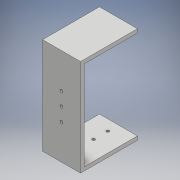
# Autodesk Inventor part: Servo Holder Upper Part
Saved by Autodesk Inventor 2018 (Build 220112000, 112)
## iProperties
Created: 2018-04-22
Part Number: Servo Holder Upper Part
Material: Generic
Document SubType Name: Modeling
Designer: HP
Density: 1 g/cm^3
Appearance: Default
Mass: 3.87293 g
Surface Area: 43.5978 cm^2
Volume: 3.87293 cm^3
Author: HP
Autodesk Inventor part; units mm, degrees
ref_plane "YZ Plane" through (0, 0, 0) normal (1, 0, 0) x (0, 1, 0)
ref_plane "XZ Plane" through (0, 0, 0) normal (0, 1, 0) x (-1, 0, 0)
ref_plane "XY Plane" through (0, 0, 0) normal (0, 0, 1) x (1, 0, 0)
sketch "Sketch9" plane through (0, 0, 0) normal (0, 1, 0) x (-1, 0, 0)
  line L0 (0, 0) -> (-20, 0)
  line L1 (-20, 0) -> (-20, -47)
  line L2 (-20, -47) -> (0, -47)
  line L3 (0, -47) -> (0, 0)
  dimension "d20" = 20
  dimension "d21" = 47
  constraints: 8 end point, 2 parallel, 1 horizontal, 1 perpendicular
  measures "d20" distance of L2.end L1.end
  measures "d21" distance of L1.end L0.end
extrude "Extrusion6" add sketch "Sketch9" along normal blind 2
sketch "Sketch10" plane through (0, 0, 0) normal (0, 0, 1) x (1, 0, 0)
  line L0 (0, 0) -> (20, 0) projected
  line L1 (0, 0) -> (20, 0)
  line L2 (20, 0) -> (20, 30)
  line L3 (20, 30) -> (0, 30)
  line L4 (0, 30) -> (0, 0)
  dimension "d24" = 30
  dimension "d40" = 20
  constraints: 8 end point, 2 parallel, 1 horizontal, 1 perpendicular
  measures "d24" distance of L2.end L1.end
  measures "d40" distance between parallel lines of L2 L4
extrude "Extrusion7" add sketch "Sketch10" along normal blind 2
sketch "Sketch11" plane through (20, 0, -47) normal (0, 0, -1) x (-1, 0, 0)
  line L0 (0, 2) -> (0, 30) projected
  line L1 (0, 0) -> (20, 0) projected
  line L2 (0, 30) -> (20, 30)
  line L3 (20, 30) -> (20, 0)
  line L4 (20, 0) -> (0, 0)
  line L5 (0, 0) -> (0, 30)
  dimension "d39" = 30
  constraints: 8 end point, 2 parallel, 1 horizontal, 1 perpendicular
  measures "d39" distance between parallel lines of L2 L1
extrude "Extrusion8" add sketch "Sketch11" along normal blind 2
sketch "Sketch12" plane through (20, 0, -49) normal (0, 0, -1) x (-1, 0, 0)
  circle A0 centre (10, 24.36) radius 0.75
  line L0 (20, 30) -> (0, 30) projected
  line L1 (0, 30) -> (0, 0) projected
  point P0 (20, 0)
  dimension "d29" = 1.5
  dimension "d30" = 5.64
  dimension "d31" = 10
  constraints: 1 centre point
  measures "d29" diameter of A0
  measures "d30" distance from line of L0 A0.centre
  measures "d31" distance from line of L1 A0.centre
extrude "Extrusion9" cut sketch "Sketch12" against normal blind 2
sketch "Sketch13" plane through (20, 0, -49) normal (0, 0, -1) x (-1, 0, 0)
  circle A0 centre (10, 16.86) radius 0.75
  line L0 (0, 30) -> (0, 0) projected
  circle A1 centre (10, 24.36) radius 0.75 projected
  point P0 (20, 0)
  dimension "d34" = 1.5
  dimension "d35" = 10
  dimension "d36" = 7.5
  constraints: 1 centre point
  measures "d34" diameter of A0
  measures "d35" distance from line of L0 A0.centre
  measures "d36" distance of A1.centre A0.centre
extrude "Extrusion10" cut sketch "Sketch13" against normal blind 2 contours A0
sketch "Sketch14" plane through (0, 0, 0) normal (0, -1, 0) x (1, 0, 0)
  circle A0 centre (10, -23.5) radius 0.75
  line L0 (0, 2) -> (0, -49) projected
  line L1 (20, -47) -> (0, -47) projected
  circle A1 centre (10, -30.6) radius 0.75
  circle A2 centre (10, -16.4) radius 0.75
  point P0 (0, 0)
  dimension "d41" = 1.5
  dimension "d42" = 10
  dimension "d43" = 23.5
  dimension "d44" = 1.5
  dimension "d45" = 7.1
  dimension "d46" = 1.5
  dimension "d47" = 7.1
  constraints: 3 centre point
  measures "d41" diameter of A0
  measures "d42" distance from line of L0 A0.centre
  measures "d43" distance from line of L1 A0.centre
  measures "d44" diameter of A1
  measures "d45" distance of A0.centre A1.centre
  measures "d46" diameter of A2
  measures "d47" distance of A2.centre A0.centre
extrude "Extrusion11" cut sketch "Sketch14" against normal blind 10
body "Solid2"
